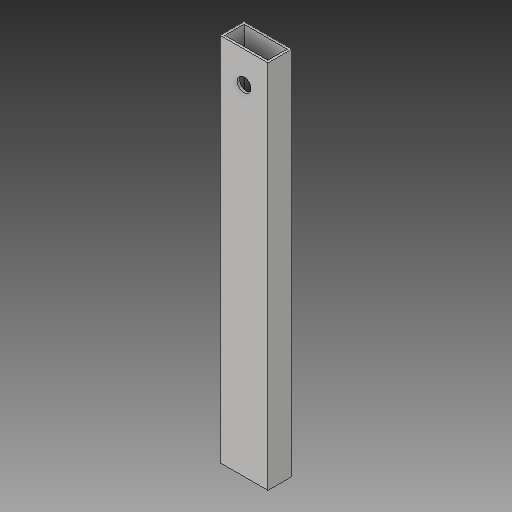
# Autodesk Inventor part: Aluminum channel pivot mount
Saved by Autodesk Inventor 2019 (Build 230136000, 136)
## iProperties
Created: 2019-03-18
Part Number: Aluminum channel pivot mount
Material: Generic
Document SubType Name: Modeling
Designer: josh
Density: 1 g/cm^3
Appearance: Default
Mass: 141.382 g
Surface Area: 1122.81 cm^2
Volume: 141.382 cm^3
Author: josh
Autodesk Inventor part; units mm, degrees
ref_plane "YZ Plane" through (0, 0, 0) normal (1, 0, 0) x (0, 1, 0)
ref_plane "XZ Plane" through (0, 0, 0) normal (0, 1, 0) x (-1, 0, 0)
ref_plane "XY Plane" through (0, 0, 0) normal (0, 0, 1) x (1, 0, 0)
sketch "Sketch1" plane through (0, 0, 0) normal (0, 1, 0) x (-1, 0, 0)
  line L0 (0, 0) -> (50.8, 0)
  line L1 (50.8, 0) -> (50.8, -25.4)
  line L2 (50.8, -25.4) -> (0, -25.4)
  line L3 (0, -25.4) -> (0, 0)
  line L4 (2.54, -22.86) -> (48.26, -22.86)
  line L5 (48.26, -22.86) -> (48.26, -2.54)
  line L6 (48.26, -2.54) -> (2.54, -2.54)
  line L7 (2.54, -2.54) -> (2.54, -22.86)
  dimension "d0" = 50.8
  dimension "d1" = 25.4
  dimension "d2" = 2.54
  constraints: 16 end point, 4 parallel, 2 perpendicular, 1 horizontal, 3 other
  measures "d0" distance of L1.end L2.end
  measures "d1" distance of L0.end L1.end
  measures "d2" distance between parallel lines of L2 L4
extrude "Extrusion1" add sketch "Sketch1" against normal blind 393.7
sketch "Sketch2" plane through (-50.8, 0, 0) normal (0, 0, 1) x (1, 0, 0)
  circle A0 centre (25.4, -32.7323) radius 7.3323 projected
  line L0 (50.8, -279.4) -> (0, -279.4) projected
  line L1 (50.8, -279.4) -> (50.8, 0) projected
  line L2 (0, 0) -> (50.8, 0) projected
  line L3 (0, -279.4) -> (0, 0) projected
  circle A1 centre (25.4, -32.7323) radius 7.3323
  constraints: 1 centre point, 1 coincident, 1 concentric
extrude "Extrusion2" cut sketch "Sketch2" against normal through all contours A0
body "Solid1"
